Autodesk Fusion 360 part; units mm, degrees
(part 2 of 2)
  constraint parallel L250 L251
  constraint coincident L74 L252.start
  constraint coincident L61 L252.end
  constraint coincident L91 L253.start
  constraint coincident L67 L253.end
  constraint parallel L252 L253
  constraint coincident L67 L254.start
  constraint coincident L91 L254.end
  constraint parallel L253 L254
  constraint coincident L67 L255.start
  constraint coincident L91 L255.end
  constraint parallel L254 L255
  constraint parallel L251 L252
  constraint midpoint L250 L256.start
  constraint midpoint L251 L256.end
  constraint midpoint L252 L257.end
  constraint midpoint L255 L258.end
  constraint midpoint L254 L259.end
  constraint midpoint L253 L260.end
  constraint equal L256 L262
  constraint equal L256 L257
  constraint equal L260 L261
  constraint equal L259 L260
  constraint equal L258 L259
  constraint equal L257 L258
  measures "d158" distance of L16.start L16.end
  measures "d159" angle of L71 L147
  measures "d164" angle of L74 L250
sketch "Sketch1 (9)" plane through (0, 0, 8.6) normal (0, 0, 1) x (-1, 0, 0) in component "SwitchPlate"
  circle A0 centre (-131, -153.5) radius 1.6
  circle A1 centre (131, 153.5) radius 1.6
  line L0 (48, 101.858) -> (-48, 101.858)
  line L1 (-48, 101.858) -> (-48, 153.858)
  line L2 (-48, 153.858) -> (48, 153.858)
  line L3 (48, 153.858) -> (48, 101.858)
  circle A2 centre (-131, 153.5) radius 1.6
  line L4 (62.5, 140.358) -> (87.5, 140.358)
  line L5 (87.5, 140.358) -> (87.5, 115.358)
  line L6 (87.5, 115.358) -> (62.5, 115.358)
  line L7 (62.5, 115.358) -> (62.5, 140.358)
  line L8 (135.6, -158.1) -> (135.6, 158.1)
  line L9 (135.6, 158.1) -> (-135.6, 158.1)
  line L10 (-135.6, 158.1) -> (-135.6, -158.1)
  line L11 (-135.6, -158.1) -> (135.6, -158.1)
  line L12 (87.5, 115.358) -> (62.5, 140.358) construction
  line L13 (87.5, 140.358) -> (62.5, 115.358) construction
  line L14 (83, 119.858) -> (67, 119.858)
  line L15 (67, 119.858) -> (67, 135.858)
  line L16 (67, 135.858) -> (83, 135.858)
  line L17 (83, 135.858) -> (83, 119.858)
  line L18 (83, 119.858) -> (67, 135.858) construction
  line L19 (67, 119.858) -> (83, 135.858) construction
  line L20 (62.65, 140.208) -> (87.35, 140.208)
  line L21 (87.35, 140.208) -> (87.35, 115.508)
  line L22 (87.35, 115.508) -> (62.65, 115.508)
  line L23 (62.65, 115.508) -> (62.65, 140.208)
  circle A3 centre (131, -153.5) radius 1.6
  point P0 (75, 127.858)
  point P1 (75, 127.858)
  point P2 (75, 127.858)
  dimension "d258" = 16
  dimension "d259" = 16
  dimension "d268" = 0.15
  constraint coincident L5.end L6.start
  constraint coincident L4.start L7.end
  constraint coincident L4.end L5.start
  constraint coincident L6.end L7.start
  constraint midpoint L12 P2
  constraint coincident P2 P1
  constraint horizontal L14
  constraint perpendicular L14 L15
  constraint parallel L14 L16
  constraint parallel L15 L17
  constraint coincident L18 P2
  constraint coincident L19 P2
  measures "d258" distance of L15.end L16.end
  measures "d259" distance of L14.end L15.end
extrude "Extrude1''''''''" add sketch "Sketch1 (9)" along normal blind 4 separate body contours L20 L21 L22 L23 makes body 9 in component "SwitchPlate"
sketch "Sketch6 (2)" plane through (0, 0, 12.6) normal (0, 0, 1) x (-1, 0, 0) in component "SwitchPlate"
  line L0 (67, 135.858) -> (83, 135.858)
  line L1 (83, 135.858) -> (83, 119.858)
  line L2 (83, 119.858) -> (67, 119.858)
  line L3 (67, 119.858) -> (67, 135.858)
  line L4 (62.65, 115.508) -> (87.35, 115.508)
  line L5 (87.35, 115.508) -> (87.35, 140.208)
  line L6 (87.35, 140.208) -> (62.65, 140.208)
  line L7 (62.65, 140.208) -> (62.65, 115.508)
  line L8 (83, 119.858) -> (67, 135.858) construction
  line L9 (83, 135.858) -> (67, 119.858) construction
  line L10 (82.025, 120.833) -> (67.975, 120.833)
  line L11 (67.975, 120.833) -> (67.975, 134.883)
  line L12 (67.975, 134.883) -> (82.025, 134.883)
  line L13 (82.025, 134.883) -> (82.025, 120.833)
  line L14 (82.025, 120.833) -> (67.975, 134.883) construction
  line L15 (67.975, 120.833) -> (82.025, 134.883) construction
  point P0 (75, 127.858)
  point P1 (75, 127.858)
  dimension "d269" = 14.05
  dimension "d270" = 14.05
  constraint coincident L1.end L2.start
  constraint coincident L0.start L3.end
  constraint coincident L0.end L1.start
  constraint coincident L2.end L3.start
  constraint midpoint L9 P1
  constraint horizontal L10
  constraint perpendicular L10 L11
  constraint parallel L10 L12
  constraint parallel L11 L13
  constraint coincident L14 P1
  constraint coincident L15 P1
  constraint coincident P1 P0
  measures "d269" distance of L11.end L12.end
  measures "d270" distance of L10.end L11.end
extrude "Extrude5" add sketch "Sketch6 (2)" against normal blind 0.5 contours L0 L1 L2 L3 bodies 9 in component "SwitchPlate"
extrude "Extrude6'" add sketch "Sketch6 (2)" along normal blind 1 contours L0 L1 L2 L3 | L4 L5 L6 L7 bodies 9 in component "SwitchPlate"
sketch "Sketch3 (3)" plane through (0, 0, 4) normal (0, 0, 1) x (-1, 0, 0) in component "PCB"
  circle A0 centre (37.7, 143.558) radius 1.4
  circle A1 centre (37.7, 112.158) radius 1.4
  circle A2 centre (-37.7, 112.158) radius 1.4
  circle A3 centre (-37.7, 143.558) radius 1.4
  line L0 (-35.35, 139.758) -> (35.35, 139.758)
  line L1 (35.35, 139.758) -> (35.35, 115.958)
  line L2 (35.35, 115.958) -> (-35.35, 115.958)
  line L3 (-35.35, 115.958) -> (-35.35, 139.758)
  line L4 (40, 145.858) -> (-40, 145.858)
  line L5 (-40, 145.858) -> (-40, 109.858)
  line L6 (-40, 109.858) -> (40, 109.858)
  line L7 (40, 109.858) -> (40, 145.858)
  line L8 (-35.35, 118.958) -> (-39.9, 123.858)
  line L9 (-39.9, 123.858) -> (-39.9, 127.858)
  line L10 (-40, 127.858) -> (-35.35, 127.858) construction
  line L11 (-35.35, 136.758) -> (-39.9, 131.858)
  line L12 (-39.9, 131.858) -> (-39.9, 127.858)
  dimension "d282" = 3
  dimension "d283" = 0.1
  dimension "d284" = 4
  constraint coincident L3 L8.start
  constraint parallel L3 L9
  constraint midpoint L5 L10.start
  constraint coincident L3 L10.end
  constraint midpoint L3 L10.end
  constraint coincident L9.end L10
  constraint symmetric L8.start L10 L11.start
  constraint symmetric L8.end L10 L11.end
  constraint symmetric L9.end L10 L12.end
  measures "d282" distance of L2.end L8.start
  measures "d283" distance of L5 L8.end
  measures "d284" distance of L8.end L9.end
extrude "Extrude5'" add sketch "Sketch3 (3)" along normal blind 3 contours L3 L8 L9 L11 L12 bodies 1 in component "PCB"
sketch "Sketch1 (10)" plane through (0, 0, 11) normal (0, 0, 1) x (-1, 0, 0) in component "ScreenCover"
  line L0 (35.35, 139.758) -> (-35.35, 139.758)
  line L1 (-35.35, 139.758) -> (-35.35, 115.958)
  line L2 (-35.35, 115.958) -> (35.35, 115.958)
  line L3 (35.35, 115.958) -> (35.35, 139.758)
  line L4 (40, 145.858) -> (-40, 145.858)
  line L5 (-40, 145.858) -> (-40, 109.858)
  line L6 (-40, 109.858) -> (40, 109.858)
  line L7 (40, 109.858) -> (40, 145.858)
  line L8 (-35.35, 118.958) -> (-39.9, 123.858)
  line L9 (-39.9, 123.858) -> (-39.9, 131.858)
  line L10 (-39.9, 131.858) -> (-35.35, 136.758)
  line L11 (-35.35, 136.758) -> (-35.35, 139.758)
  line L12 (-35.35, 139.758) -> (35.35, 139.758)
  line L13 (35.35, 139.758) -> (35.35, 115.958)
  line L14 (35.35, 115.958) -> (-35.35, 115.958)
  line L15 (-35.35, 115.958) -> (-35.35, 118.958)
  circle A0 centre (-37.7, 143.558) radius 1.4
  circle A1 centre (-37.7, 112.158) radius 1.4
  circle A2 centre (37.7, 112.158) radius 1.4
  circle A3 centre (37.7, 143.558) radius 1.4
  line L16 (62.5, 140.358) -> (87.5, 140.358)
  line L17 (87.5, 140.358) -> (87.5, 115.358)
  line L18 (87.5, 115.358) -> (62.5, 115.358)
  line L19 (62.5, 115.358) -> (62.5, 140.358)
  line L20 (48, 101.858) -> (-48, 101.858)
  line L21 (-48, 101.858) -> (-48, 153.858)
  line L22 (-48, 153.858) -> (48, 153.858)
  line L23 (48, 153.858) -> (48, 101.858)
  circle A4 centre (131, 153.5) radius 1.6
  circle A5 centre (-131, -153.5) radius 1.6
  circle A6 centre (-131, 153.5) radius 1.6
  line L24 (135.6, -158.1) -> (135.6, 158.1)
  line L25 (135.6, 158.1) -> (-135.6, 158.1)
  line L26 (-135.6, 158.1) -> (-135.6, -158.1)
  line L27 (-135.6, -158.1) -> (135.6, -158.1)
  line L28 (35.85, 140.258) -> (-35.85, 140.258)
  line L29 (-35.85, 140.258) -> (-35.85, 115.458)
  line L30 (-35.85, 115.458) -> (35.85, 115.458)
  line L31 (35.85, 115.458) -> (35.85, 140.258)
  line L32 (-47.5, 153.358) -> (47.5, 153.358)
  line L33 (47.5, 153.358) -> (47.5, 102.358)
  line L34 (47.5, 102.358) -> (-47.5, 102.358)
  line L35 (-47.5, 102.358) -> (-47.5, 153.358)
  circle A7 centre (-37.7, 143.558) radius 1.6
  circle A8 centre (37.7, 143.558) radius 1.6
  circle A9 centre (37.7, 112.158) radius 1.6
  circle A10 centre (-37.7, 112.158) radius 1.6
  circle A11 centre (131, -153.5) radius 1.6
  dimension "d287" = 0.5
  dimension "d288" = 0.5
  dimension "d307" = 3.2
  constraint concentric A0 A7
  constraint concentric A3 A8
  constraint concentric A2 A9
  constraint concentric A1 A10
  constraint equal A9 A10
  constraint equal A8 A9
  constraint equal A7 A8
  measures "d307" diameter of A7
extrude "Extrude1'''''''''" add sketch "Sketch1 (10)" against normal blind 7 separate body contours L8 L9 L10 L29 | L4 L5 L6 L7 | L32 L33 L34 L35 makes body 10 in component "ScreenCover"
sketch "Sketch2 (3)" plane through (0, 0, 4) normal (0, 0, -1) x (1, 0, 0) in component "ScreenCover"
  line L0 (-35.85, 115.458) -> (-35.85, 140.258)
  line L1 (-35.85, 140.258) -> (35.85, 140.258)
  line L2 (35.85, 140.258) -> (35.85, 115.458)
  line L3 (35.85, 115.458) -> (-35.85, 115.458)
  line L4 (-47.5, 102.358) -> (47.5, 102.358)
  line L5 (47.5, 102.358) -> (47.5, 153.358)
  line L6 (47.5, 153.358) -> (-47.5, 153.358)
  line L7 (-47.5, 153.358) -> (-47.5, 102.358)
  line L8 (35.35, 118.958) -> (35.35, 136.758)
  line L9 (35.35, 136.758) -> (39.9, 131.858)
  line L10 (39.9, 131.858) -> (39.9, 123.858)
  line L11 (39.9, 123.858) -> (35.35, 118.958)
  line L12 (41.9, 123.0726) -> (33.35, 113.8649)
  line L13 (33.35, 113.8649) -> (33.35, 141.8511)
  line L14 (33.35, 141.8511) -> (41.9, 132.6434)
  line L15 (41.9, 132.6434) -> (41.9, 123.0726)
  line L16 (-33.7, 115.658) -> (16.3, 115.658)
  line L17 (16.3, 115.658) -> (16.3, 108.658)
  line L18 (16.3, 108.658) -> (-33.7, 108.658)
  line L19 (-33.7, 108.658) -> (-33.7, 115.658)
  circle A0 centre (37.7, 143.558) radius 1.6
  circle A1 centre (-37.7, 143.558) radius 1.6
  circle A2 centre (37.7, 112.158) radius 1.6
  circle A3 centre (-37.7, 112.158) radius 1.6
  line L20 (-33.7, 112.158) -> (-37.7, 112.158) construction
  dimension "d291" = -2
  dimension "d296" = 7
  dimension "d297" = 50
  dimension "d319" = 4
  constraint horizontal L16
  constraint vertical L17
  constraint horizontal L18
  constraint vertical L19
  constraint midpoint L19 L20.start
  constraint perpendicular L19 L20
  constraint coincident A3.centre L20.end
  measures "d296" distance of L16.end L17.end
  measures "d297" distance of L16.start L16.end
  measures "d319" distance of L20.start A3.centre
extrude "Extrude2''" cut sketch "Sketch2 (3)" against normal blind 5 contours L2 L9 L10 L11 L12 L14 L15 | L2 L9 L10 L11 bodies 10 in component "ScreenCover"
extrude "Extrude3''" cut sketch "Sketch2 (3)" against normal blind 2.5 contours L3 L16 L17 L19 | L3 L17 L18 L19 bodies 10 in component "ScreenCover"
sketch "Sketch1 (11)" plane through (0, -13.8, 0) normal (0, -1, 0) x (1, 0, 0) in component "Brace"
  circle A0 centre (121.8, -35.5) radius 1.45
  circle A1 centre (121.8, -5.5) radius 1.45
  line L0 (117.2, -40) -> (135.6, -40)
  line L1 (135.6, -40) -> (135.6, -1)
  line L2 (135.6, -1) -> (117.2, -1)
  line L3 (117.2, -1) -> (117.2, -40)
  circle A2 centre (-121.8, -35.5) radius 1.45
  circle A3 centre (-121.8, -5.5) radius 1.45
  line L4 (-135.6, -40) -> (-117.2, -40)
  line L5 (-117.2, -40) -> (-117.2, -1)
  line L6 (-117.2, -1) -> (-135.6, -1)
  line L7 (-135.6, -1) -> (-135.6, -40)
  line L8 (36.3, 0) -> (39.1, 0)
  line L9 (36.3, 0) -> (39.1, 0)
  line L10 (-39.1, 0) -> (-36.3, 0)
  line L11 (-39.1, 0) -> (-36.3, 0)
  line L12 (-132.6, 0) -> (-129.4, 0)
  line L13 (122.64, 0) -> (112.36, 0)
  line L14 (112.36, 0) -> (122.64, 0)
  line L15 (129.4, 0) -> (132.6, 0)
  line L16 (-132.6, 0) -> (-129.4, 0)
  line L17 (129.4, 0) -> (132.6, 0)
  line L18 (135, 0) -> (-135, 0)
  line L19 (-135, 0) -> (135, 0)
  line L20 (-135.6, -1) -> (-135.6, 0)
  line L21 (-135.6, 0) -> (-135, 0)
  line L22 (135, 0) -> (135.6, 0)
  line L23 (135.6, 0) -> (135.6, -1)
  line L24 (117.2, -40) -> (-117.2, -40)
  constraint coincident L6.end L7.start
  constraint perpendicular L6 L20
  constraint coincident L18.end L19.start
  constraint perpendicular L20 L21
  constraint coincident L18.start L19.end
  constraint parallel L19 L22
  constraint coincident L1.end L2.start
  constraint perpendicular L22 L23
  constraint coincident L0.start L3.end
  constraint coincident L4.end L5.start
extrude "Extrude1''''''''''" add sketch "Sketch1 (11)" along normal blind 3 separate body makes body 11 in component "Brace"
sketch "Sketch2 (4)" plane through (0, -161.1, 0) normal (0, -1, 0) x (1, 0, 0) in component "Panel1"
  circle A0 centre (121.8, -35.5) radius 1.6
  circle A1 centre (121.8, -5.5) radius 1.6
  circle A2 centre (-121.8, -35.5) radius 1.6
  circle A3 centre (-121.8, -5.5) radius 1.6
  line L0 (-135.6, 8.6) -> (-135.6, -40)
  line L1 (-135.6, -40) -> (135.6, -40)
  line L2 (135.6, -40) -> (135.6, 8.6)
  line L3 (135.6, 8.6) -> (-135.6, 8.6)
  circle A4 centre (121.8, -35.5) radius 1.6
  circle A5 centre (121.8, -5.5) radius 1.6
  circle A6 centre (-121.8, -35.5) radius 1.6
  circle A7 centre (-121.8, -5.5) radius 1.6
  line L4 (-135.6, 8.6) -> (-135.6, -40)
  line L5 (-135.6, -40) -> (135.6, -40)
  line L6 (135.6, -40) -> (135.6, 8.6)
  line L7 (135.6, 8.6) -> (-135.6, 8.6)
sketch "Sketch2 (5)" plane through (138.6, 0, 0) normal (1, 0, 0) x (0, 1, 0) in component "Panel2"
  circle A0 centre (0, -5.5) radius 1.6
  circle A1 centre (0, -35.5) radius 1.6
  circle A2 centre (144.3, -5.5) radius 1.6
  circle A3 centre (-144.3, -35.5) radius 1.6
  circle A4 centre (-144.3, -5.5) radius 1.6
  circle A5 centre (144.3, -35.5) radius 1.6
  line L0 (-119.02, 8.6) -> (-119.02, -2.4)
  line L1 (-119.02, -2.4) -> (-136.02, -2.4)
  line L2 (-136.02, -2.4) -> (-136.02, 8.6)
  line L3 (-136.02, 8.6) -> (-161.1, 8.6)
  line L4 (-161.1, 8.6) -> (-161.1, -40)
  line L5 (-161.1, -40) -> (161.1, -40)
  line L6 (161.1, -40) -> (161.1, 8.6)
  line L7 (161.1, 8.6) -> (-119.02, 8.6)
sketch "Sketch2 (6)" plane through (-138.6, 0, 0) normal (-1, 0, 0) x (0, -1, 0) in component "Panel3"
  circle A0 centre (144.3, -5.5) radius 1.6
  circle A1 centre (-144.3, -35.5) radius 1.6
  circle A2 centre (-144.3, -5.5) radius 1.6
  circle A3 centre (144.3, -35.5) radius 1.6
  circle A4 centre (0, -5.5) radius 1.6
  circle A5 centre (0, -35.5) radius 1.6
  line L0 (161.1, 8.6) -> (-161.1, 8.6)
  line L1 (-161.1, 8.6) -> (-161.1, -40)
  line L2 (-161.1, -40) -> (161.1, -40)
  line L3 (161.1, -40) -> (161.1, 8.6)
sketch "Sketch2 (7)" plane through (0, -16.8, 0) normal (0, -1, 0) x (1, 0, 0) in component "Brace"
  circle A0 centre (-121.8, -5.5) radius 1.45
  circle A1 centre (-121.8, -35.5) radius 1.45
  circle A2 centre (121.8, -5.5) radius 1.45
  circle A3 centre (121.8, -35.5) radius 1.45
  line L0 (135.6, -40) -> (135.6, 0)
  line L1 (135.6, 0) -> (-135.6, 0)
  line L2 (-135.6, 0) -> (-135.6, -40)
  line L3 (-135.6, -40) -> (135.6, -40)
component "PCB" placed x (1, 0, 0) y (0, 1, 0) z (0, 0, 1) at (0, 0, 0)
component "Connectors" placed x (1, 0, 0) y (0, 1, 0) z (0, 0, 1) at (0, 0, 0)
component "Hardware" placed x (1, 0, 0) y (0, 1, 0) z (0, 0, 1) at (0, 0, 0)
component "Panels" placed x (1, 0, 0) y (0, 1, 0) z (0, 0, 1) at (0, 0, 0)
component "SwitchPlate" placed x (1, 0, 0) y (0, 1, 0) z (0, 0, 1) at (0.15, -0.15, -7)
component "ScreenCover" placed x (1, 0, 0) y (0, 1, 0) z (0, 0, 1) at (0, 0, 0)
component "Corner" placed x (1, 0, 0) y (0, 1, 0) z (0, 0, 1) at (-131, 153.5, -10) in component "Connectors"
component "Washer" placed x (0, -1, 0) y (1, 0, 0) z (0, 0, 1) at (131, 153.5, -1) in component "Connectors"
component "PlateWasher" placed x (1, 0, 0) y (0, 1, 0) z (0, 0, 1) at (-131, -153.5, 1.6) in component "Connectors"
component "Corner" placed x (0, -1, 0) y (1, 0, 0) z (0, 0, 1) at (131, 153.5, -10) in component "Connectors"
component "Corner" placed x (-1, 0, 0) y (0, -1, 0) z (0, 0, 1) at (131, -153.5, -10) in component "Connectors"
component "Corner" placed x (0, 1, 0) y (-1, 0, 0) z (0, 0, 1) at (-131, -153.5, -10) in component "Connectors"
component "Washer" placed x (0, 1, 0) y (-1, 0, 0) z (0, 0, 1) at (-131, -153.5, -1) in component "Connectors"
component "Washer" placed x (1, 0, 0) y (0, 1, 0) z (0, 0, 1) at (-131, 153.5, -1) in component "Connectors"
component "Washer" placed x (-1, 0, 0) y (0, -1, 0) z (0, 0, 1) at (131, -153.5, -1) in component "Connectors"
component "PlateWasher" placed x (1, 0, 0) y (0, 1, 0) z (0, 0, 1) at (131, 153.5, 1.6) in component "Connectors"
component "PlateWasher" placed x (1, 0, 0) y (0, 1, 0) z (0, 0, 1) at (-131, 153.5, 1.6) in component "Connectors"
component "PlateWasher" placed x (1, 0, 0) y (0, 1, 0) z (0, 0, 1) at (131, -153.5, 1.6) in component "Connectors"
component "Corner" placed x (0, 1, 0) y (-1, 0, 0) z (0, 0, 1) at (-131, -9.2, -10) in component "Connectors"
component "Corner" placed x (-1, 0, 0) y (0, -1, 0) z (0, 0, 1) at (131, -9.2, -10) in component "Connectors"
component "Panel1" placed x (1, 0, 0) y (0, 1, 0) z (0, 0, 1) at (0, 319.2, 0) in component "Panels"
component "Panel1" placed x (1, 0, 0) y (0, 1, 0) z (0, 0, 1) at (0, 0, 0) in component "Panels"
component "Panel2" placed x (1, 0, 0) y (0, 1, 0) z (0, 0, 1) at (0, 0, 0) in component "Panels"
component "Panel3" placed x (1, 0, 0) y (0, 1, 0) z (0, 0, 1) at (0, 0, 0) in component "Panels"
component "TopPanel" placed x (1, 0, 0) y (0, 1, 0) z (0, 0, 1) at (0, 0, 0) in component "Panels"
component "Brace" placed x (1, 0, 0) y (0, 1, 0) z (0, 0, 1) at (0, 0, 0) in component "Panels"
equation "BoltHoleDiameter = 3.2 mm"
equation "HeatInsertDiameter = 4.6 mm"
equation "HeatInsertLength = 6 mm"
equation "PCBToPlate = 4 mm" comment "Distance from top of PCB to the bottom of plate"
equation "MaterialThickness = 3 mm" comment "Laser cut material thickness"
equation "d36 = 11 mm - 7 mm"
equation "WasherThickness = 1 mm" comment "Must be multiple of PCBToPlate"
equation "d41 = HeatInsertDiameter"
equation "d42 = HeatInsertDiameter * 2"
equation "d43 = HeatInsertDiameter"
equation "d44 = HeatInsertDiameter"
equation "d45 = HeatInsertLength + 3 mm"
equation "d49 = BoltThreadHoleDiameter"
equation "d50 = -HeatInsertLength"
equation "d52 = BoltThreadHoleDiameter"
equation "d53 = -HeatInsertLength"
equation "d55 = BoltHoleDiameter"
equation "d57 = WasherThickness"
equation "d59 = BoltHoleDiameter"
equation "d61 = PCBToPlate"
equation "d120 = MaterialThickness"
equation "d121 = MaterialThickness"
equation "d123 = BoltHoleDiameter"
equation "d129 = BoltHoleDiameter"
equation "d130 = MaterialThickness"
equation "d132 = MaterialThickness"
equation "d134 = MaterialThickness"
equation "d236 = PCBToPlate"
equation "d253 = 5 mm - PCBToPlate - 1.5 mm"
equation "d256 = 5 mm - PCBToPlate"
equation "d274 = -PCBToPlate"
equation "BoltThreadHoleDiameter = 2.9 mm"
equation "d307 = BoltHoleDiameter"
equation "d316 = MaterialThickness"
